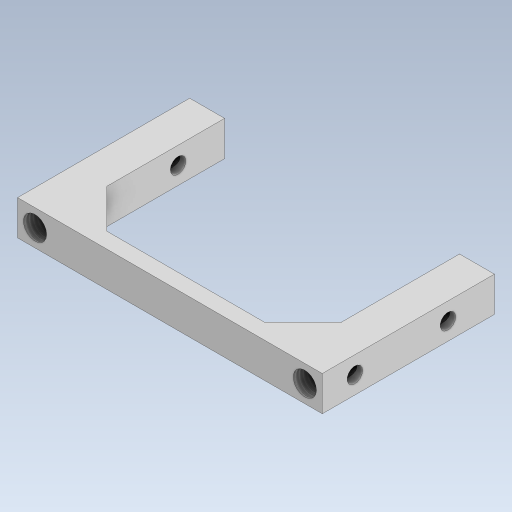
# Autodesk Inventor part: Tiang 1
Saved by Autodesk Inventor 2023.5 (Build 275446000, 446)
## iProperties
Created: 2025-09-05
Part Number: Tiang 1
Material: Generic
Document SubType Name: Modeling
Designer: Guntur
Density: 1 g/cm^3
Appearance: Default
Author: Guntur
Autodesk Inventor part; units mm, degrees
ref_plane "YZ Plane" through (0, 0, 0) normal (1, 0, 0) x (0, 1, 0)
ref_plane "XZ Plane" through (0, 0, 0) normal (0, 1, 0) x (-1, 0, 0)
ref_plane "XY Plane" through (0, 0, 0) normal (0, 0, 1) x (1, 0, 0)
sketch "Sketch1" plane through (0, 0, 0) normal (0, 0, 1) x (1, 0, 0)
  circle A0 centre (-17.4, 0) radius 1.5
  line L0 (0, 7.9375) -> (0, -7.1814) construction
  line L1 (-8.2631, 0) -> (10.6068, 0) construction
  line L2 (-19.65, 2.25) -> (-15.15, 2.25)
  line L3 (-15.15, 2.25) -> (-15.15, -2.25)
  line L4 (-15.15, -2.25) -> (-19.65, -2.25)
  line L5 (-19.65, -2.25) -> (-19.65, 2.25)
  line L6 (-19.65, 2.25) -> (-15.15, -2.25) construction
  line L7 (-15.15, 2.25) -> (-19.65, -2.25) construction
  circle A1 centre (17.4, 0) radius 1.5
  line L8 (19.65, 2.25) -> (15.15, 2.25)
  line L9 (15.15, 2.25) -> (15.15, -2.25)
  line L10 (15.15, -2.25) -> (19.65, -2.25)
  line L11 (19.65, -2.25) -> (19.65, 2.25)
  line L12 (19.65, 2.25) -> (15.15, -2.25) construction
  line L13 (15.15, 2.25) -> (19.65, -2.25) construction
  point P0 (0, 0)
  dimension "d0" = 3
  dimension "d1" = 17.4
  dimension "d2" = 4.5
  dimension "d3" = 4.5
  constraints: 28 end point, 5 symmetric about line, 2 centre point, 2 horizontal, 2 midpoint, 2 parallel, 1 perpendicular, 1 vertical, 1 other
  measures "d0" diameter of A0
  measures "d1" distance from line of L0 A0.centre
  measures "d2" distance of L3.end L4.end
  measures "d3" distance of L2.end L3.end
extrude "Extrusion1" add sketch "Sketch1" along normal blind 20.2 contours A0 | L2 L3 L4 L5 | A1 | L11 L10 L9 L8
extrude "Extrusion2" cut sketch "Sketch1" along normal blind 22.2 contours A0 | A1
ref_plane "Work Plane1" through (19.65, 0, 20.2) normal (0, 0, 1) x (1, 0, 0)
sketch "Sketch2" plane through (19.65, 0, 20.2) normal (0, 0, 1) x (1, 0, 0)
  line L0 (-39.3, 2.25) -> (-39.3, -2.25) projected
  line L1 (0, -2.25) -> (0, 2.25) projected
  line L2 (-39.3, 2.25) -> (0, 2.25)
  line L3 (0, 2.25) -> (0, -2.25)
  line L4 (0, -2.25) -> (-39.3, -2.25)
  line L5 (-39.3, -2.25) -> (-39.3, 2.25)
  point P0 (-19.65, 0)
  constraints: 8 end point, 2 parallel, 1 horizontal, 1 perpendicular
extrude "Extrusion3" add sketch "Sketch2" along normal blind 2
ref_plane "Work Plane2" through (15.15, 0, 0) normal (0, -1, 0) x (1, 0, 0)
sketch "Sketch5" plane through (15.15, 0, 0) normal (0, -1, 0) x (1, 0, 0)
  line L0 (0, 20.2) -> (-30.3, 20.2) projected
  line L1 (-30.3, 20.2) -> (-25.3, 20.2)
  line L2 (-30.3, 20.2) -> (-30.3, 15.2)
  line L3 (-30.3, 0) -> (-30.3, 20.2) projected
  line L4 (-30.3, 15.2) -> (-25.3, 20.2)
  line L5 (0, 0) -> (0, 20.2) projected
  line L6 (0, 20.2) -> (-5, 20.2)
  line L7 (-5, 20.2) -> (0, 15.2)
  line L8 (0, 15.2) -> (0, 20.2)
  point P0 (-15.15, 0)
  dimension "d10" = 5
  dimension "d11" = 5
  dimension "d12" = 5
  constraints: 12 end point, 3 point on line, 1 perpendicular
  measures "d10" distance of L0.end L1.end
  measures "d11" distance of L0.end L2.end
  measures "d12" distance of L0.start L6.end
extrude "Extrusion4" add sketch "Sketch5" along normal mid plane 4.5
sketch "Sketch6" plane through (19.65, 0, 22.2) normal (0, 0, 1) x (1, 0, 0)
  circle A0 centre (-37.05, 0) radius 1.5 projected
  circle A1 centre (-37.05, 0) radius 1.5
  circle A2 centre (-2.25, 0) radius 1.5 projected
  circle A3 centre (-2.25, 0) radius 1.5
  point P0 (-19.65, 0)
  constraints: 2 centre point, 2 coincident
extrude "Extrusion5" cut sketch "Sketch6" against normal blind 2
thread "Thread1" size "M3x0.5" class "6H" standard "ANSI Metric M Profile" full length
thread "Thread2" size "M3x0.5" class "6H" standard "ANSI Metric M Profile" full length
sketch "Sketch7" plane through (19.65, -2.25, 0) normal (1, 0, 0) x (0, 0, -1)
  circle A0 centre (-6, 2.25) radius 1
  line L0 (0, 0) -> (0, 4.5) projected
  circle A1 centre (-18, 2.25) radius 1
  point P0 (0, 2.25)
  point P1 (0, 2.25)
  dimension "d21" = 2
  dimension "d22" = 6
  dimension "d23" = 2
  dimension "d24" = 12
  constraints: 2 centre point, 1 midpoint
  measures "d21" diameter of A0
  measures "d22" distance of point (0, 2.25) A0.centre
  measures "d23" diameter of A1
  measures "d24" distance of A0.centre A1.centre
extrude "Extrusion6" cut sketch "Sketch7" against normal blind 40
body "Solid1"
